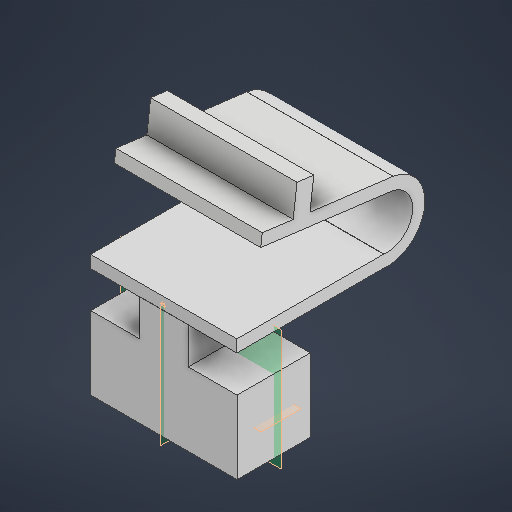
# Autodesk Inventor part: Clipper
Saved by Autodesk Inventor 2027 (Build 310192000, 192)
## iProperties
Created: 2026-03-31
Part Number: Clipper
Material: Generisch
Document SubType Name: Modeling
Designer: thomas
Density: 1 g/cm^3
Appearance: Vorgabe
Author: thomas
Autodesk Inventor part; units mm, degrees
ref_plane "YZ Plane" through (0, 0, 0) normal (1, 0, 0) x (0, 1, 0)
ref_plane "XZ Plane" through (0, 0, 0) normal (0, 1, 0) x (-1, 0, 0)
ref_plane "XY Plane" through (0, 0, 0) normal (0, 0, 1) x (1, 0, 0)
sketch "Sketch6" plane through (0, 0, 0) normal (0, 0, 1) x (1, 0, 0)
  line L0 (3, -1.5) -> (3, 1.5)
  line L1 (3, 1.5) -> (-3, 1.5)
  line L2 (-3, 1.5) -> (-3, -1.5)
  line L3 (-3, -1.5) -> (3, -1.5)
  line L4 (3, -1.5) -> (-3, 1.5) construction
  line L5 (3, 1.5) -> (-3, -1.5) construction
  point P0 (0, 0)
  dimension "d11" = 3
  dimension "d12" = 6
  constraints: 12 end point, 2 midpoint, 2 parallel, 1 perpendicular, 1 vertical
  measures "d11" distance of L0.start L0.end
  measures "d12" distance of L1.end L0.end
extrude "Extrusion4" add sketch "Sketch6" along normal mid plane 3
ref_plane "Work Plane1" through (0, 0, 0) normal (0, 0, 1) x (1, 0, 0)
sketch "Sketch8" plane through (0, 0, 1.5) normal (0, 0, 1) x (1, 0, 0)
  line L0 (-1, -1.5) -> (-1, 1.5)
  line L1 (-1, 1.5) -> (1, 1.5)
  line L2 (1, 1.5) -> (1, -1.5)
  line L3 (1, -1.5) -> (-1, -1.5)
  line L4 (-1, -1.5) -> (1, 1.5) construction
  line L5 (-1, 1.5) -> (1, -1.5) construction
  line L6 (3, 1.5) -> (-3, 1.5) projected
  point P0 (0, 0)
  dimension "d19" = 3
  dimension "d20" = 2
  constraints: 12 end point, 2 midpoint, 2 parallel, 1 collinear, 1 perpendicular
  measures "d19" distance of L0.start L0.end
  measures "d20" distance of L0.end L1.end
extrude "Extrusion6" add sketch "Sketch8" along normal blind 1.5
ref_plane "Work Plane4" through (-3, 0, -1.5) normal (0, 1, 0) x (1, 0, 0)
ref_plane "Work Plane5" through (0, -1.5, 1.5) normal (-1, 0, 0) x (0, 0, 1)
sketch "Sketch9" plane through (0, 0, 3) normal (0, 0, 1) x (1, 0, 0)
  point P0 (0, 0)
sketch "Sketch10" plane through (0, -1.5, 1.5) normal (-1, 0, 0) x (0, 0, 1)
  point P0 (-1.5, 1.5)
sketch "Sketch11" plane through (0, 0, 3) normal (0, 0, 1) x (1, 0, 0)
  point P0 (0, 0)
sketch "Sketch12" plane through (0, -1.5, 1.5) normal (-1, 0, 0) x (0, 0, 1)
  point P0 (-1.5, 1.5)
sketch "Sketch13" plane through (0, -1.5, 1.5) normal (-1, 0, 0) x (0, 0, 1)
  point P0 (-1.5, 1.5)
sketch "Sketch15" plane through (0, -1.5, 1.5) normal (-1, 0, 0) x (0, 0, 1)
  line L0 (1.75, -0.0091) -> (1.75, 5.9909)
  arc A0 (4.3235, 6.3575) -> (1.75, 5.9909) centre (3.0405, 6.1478) ccw
  line L1 (4.3235, 6.3575) -> (5, 1)
  line L2 (0, 0) -> (1.5, 0) projected
  line L3 (1.5, 0) -> (6.1638, 0) construction
  line L4 (1.5, 3) -> (1.5, 0) projected
  point P0 (-1.5, 1.5)
  dimension "d31" = 6
  dimension "d33" = 1.3
  dimension "d34" = 5.4
  dimension "d41" = 0.25
  constraints: 6 end point, 2 point on circle, 1 centre point, 1 horizontal, 1 vertical
  measures "d31" distance of L0.start L0.end
  measures "d33" radius of A0
  measures "d34" distance of L1.start L1.end
  measures "d41" distance between parallel lines of L0 L4
sketch "Sketch18" plane through (-3, -1.5, -1.5) normal (0, -1, 0) x (1, 0, 0)
  line L0 (6, 4.5) -> (0, 4.5)
  line L1 (0, 4.5) -> (0, 5)
  line L2 (0, 5) -> (6, 5)
  line L3 (6, 5) -> (6, 4.5)
  line L4 (6, 4.5) -> (0, 5) construction
  line L5 (0, 4.5) -> (6, 5) construction
  line L6 (2, 4.5) -> (4, 4.5) projected
  point P0 (3, 1.5)
  point P1 (3, 4.75)
  point P2 (3, 4.5)
  point P3 (3, 4.5)
  dimension "d37" = 6
  dimension "d38" = 0.5
  dimension "d42" = 0
  constraints: 12 end point, 4 midpoint, 2 parallel, 1 horizontal, 1 perpendicular
  measures "d37" distance of L0.start L0.end
  measures "d38" distance of L0.end L1.end
  measures "d42" distance of point (3, 4.5) point (3, 4.5)
sweep "Sweep1" add profiles "Sketch18" path "Sketch15" separate body path curves L0 A0 L1
sketch "Sketch19" plane through (-3, 4.8978, 6.0704) normal (0, 0.1252822, 0.9921211) x (1, 0, 0)
  line L0 (0, -6.0344) -> (0, -0.0667) projected
  line L1 (6, -0.0139) -> (6, -5.4091) projected
  line L2 (0, -3.4382) -> (6, -3.4382)
  line L3 (6, -3.4382) -> (6, -4.132)
  line L4 (6, -4.132) -> (0, -4.132)
  line L5 (0, -4.132) -> (0, -3.4382)
  point P0 (3, -4.0987)
  point P1 (6, -0.1471)
  point P2 (0, -4.132)
  point P3 (6, -3.4382)
  constraints: 8 end point, 2 parallel, 2 point on line, 1 horizontal, 1 perpendicular
extrude "Extrusion7" add sketch "Sketch19" along normal blind 1.25 bodies 2
equation "\"d11\" = PCB_thickness"
equation "\"d12\" = clipper_uppter_t_length"
equation "\"d13\" = 0.5 * wall_thickness"
equation "\"d19\" = PCB_thickness"
equation "\"d20\" = clipp_lower_t_part_thickness"
equation "\"d21\" = 0.25 * wall_thickness"
equation "\"d31\" = arm_heigth"
equation "\"d33\" = arc_radius"
equation "\"d34\" = 0.9 * arm_heigth"
equation "\"d41\" = 0.5 * spring_thickness"
equation "\"d37\" = spring_width"
equation "\"d38\" = spring_thickness"
equation "\"wall_thickness\" = 6"
equation "\"PCB_thickness\" = 3"
equation "\"clipp_lower_t_part_thickness\" = 2"
equation "\"clipper_uppter_t_length\" = 6"
equation "\"arm_heigth\" = 6"
equation "\"arc_radius\" = 1.3"
equation "\"gap_width\" = 2.5"
equation "\"spring_thickness\" = 0.5"
equation "\"spring_width\" = 6"
equation "\"hook_length\" = 3"
body "Solid3"
body "Solid4"
